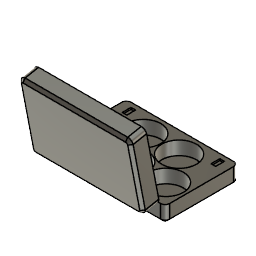
Loupe Case (Autodesk Fusion 360 design; units mm, degrees)
Autodesk Fusion 360 part; units mm, degrees
sketch "Sketch1" plane through (0, 0, 0) normal (0, 0, 1) x (1, 0, 0)
  line L0 (61, 39.8875) -> (-61, 39.8875)
  line L1 (-61, 39.8875) -> (-61, -39.8875)
  line L2 (-61, -39.8875) -> (61, -39.8875)
  line L3 (61, -39.8875) -> (61, 39.8875)
  line L4 (61, 39.8875) -> (-61, -39.8875) construction
  line L5 (-61, 39.8875) -> (61, -39.8875) construction
  line L6 (-71.3663, 44.8875) -> (78.0127, 44.8875) construction
  line L7 (61, 49.8875) -> (-61, 49.8875)
  line L8 (-61, 49.8875) -> (-61, 129.6625)
  line L9 (-61, 129.6625) -> (61, 129.6625)
  line L10 (61, 129.6625) -> (61, 49.8875)
  circle A0 centre (-39, 16.8875) radius 19
  line L11 (0, 0) -> (0, -7.9518) construction
  circle A1 centre (0, 16.8875) radius 19
  circle A2 centre (39, 16.8875) radius 19
  circle A3 centre (-19.5, -16.8875) radius 19
  line L12 (-39, 16.8875) -> (-19.5, -16.8875) construction
  line L13 (-39, 16.8875) -> (-33.2699, 16.8875) construction
  circle A4 centre (19.5, -16.8875) radius 19
  circle A5 centre (19.5, 106.6625) radius 19
  circle A6 centre (-19.5, 106.6625) radius 19
  circle A7 centre (39, 72.8875) radius 19
  circle A8 centre (0, 72.8875) radius 19
  circle A9 centre (-39, 72.8875) radius 19
  dimension "d2" = 79.775
  dimension "d3" = 10
  dimension "d6" = 38
  dimension "d10" = 39
  dimension "d11" = 0
  dimension "d12" = 3
  dimension "d13" = 1
  dimension "d15" = 4
  dimension "d17" = 60
  dimension "d18" = 1
  dimension "d19" = 4
  constraint horizontal L0
  constraint perpendicular L0 L1
  constraint parallel L0 L2
  constraint parallel L1 L3
  constraint coincident L4 L11.start
  constraint coincident L5 L11.start
  constraint coincident L11.start origin
  constraint parallel L0 L6
  constraint symmetric L0.start L6 L7.start
  constraint symmetric L0.end L6 L7.end
  constraint symmetric L1.end L6 L8.end
  constraint symmetric L2.end L6 L9.end
  constraint vertical L11
  constraint vertical L11.start A1.centre
  constraint equal A0 A3
  constraint coincident A0.centre L12.start
  constraint horizontal L13
  constraint coincident A3.centre L12.end
  constraint symmetric L11 A3 A4
  constraint symmetric L6 A0 A9
  constraint symmetric L6 A1 A8
  constraint symmetric L6 A2 A7
  constraint symmetric L6 A3 A6
  constraint symmetric L6 A4 A5
  measures "d2" distance of L0.end L1.end
  measures "d3" distance of L0 L7
  measures "d6" diameter of A0
  measures "d12" distance of L1 A0
  measures "d13" distance of A0 A1
  measures "d15" distance of L0 A0
  measures "d17" angle of L12 L13
  measures "d18" distance of A0 A3
  measures "d19" distance of L2 A3
extrude "Extrude1" add sketch "Sketch1" along normal blind 18 contours L0 L1 L2 L3 | L7 L8 L9 L10 | A0 | A1 | A2 | A3 | A4 | A5 | A6 | A7 | A8 | A9 makes body 1 at (-20.3333, 103.0708, 0) makes body 2 at (-20.3333, 13.2958, 0)
extrude "Extrude2" cut sketch "Sketch1" against normal blind 15 from surface at 18 contours A0 | A1 | A2 | A3 | A4 | A5 | A6 | A7 | A8 | A9 bodies 1 2
sketch "Sketch2" plane through (61, 0, 0) normal (1, 0, 0) x (0, 1, 0)
  line L0 (-39.8875, 0) -> (39.8875, 0)
  line L1 (39.8875, 0) -> (39.8875, 18)
  line L2 (39.8875, 18) -> (-39.8875, 18)
  line L3 (-39.8875, 18) -> (-39.8875, 0)
  line L4 (39.8875, 0) -> (39.8875, 18)
  line L5 (39.8875, 18) -> (39.8875, 0)
  line L6 (49.8875, 0) -> (49.8875, 18)
  line L7 (49.8875, 18) -> (49.8875, 0)
  line L8 (39.8875, 7.3431) -> (47.7159, 15.1716)
  line L9 (49.8875, 7.3431) -> (42.0591, 15.1716)
  line L10 (39.8875, 18) -> (49.8875, 18) construction
  circle A0 centre (44.8875, 18) radius 4
  line L11 (39.8875, 18) -> (40.8875, 18)
  line L12 (49.8875, 18) -> (48.8875, 18)
  dimension "d23" = 135
  dimension "d24" = 135
  dimension "d25" = 1
  constraint coincident L5 L8.start
  constraint coincident L6 L9.start
  constraint coincident L1.end L2.start
  constraint coincident L6.end L7.start
  constraint midpoint L10 A0.centre
  constraint coincident L8.end A0
  constraint tangent L8 A0
  constraint coincident L9.end A0
  constraint tangent L9 A0
  constraint coincident A0 L11.end
  constraint coincident L10 L11.end
  constraint coincident A0 L12.end
  constraint coincident L10 L12.end
  measures "d23" angle of L5 L8
  measures "d24" angle of L6 L9
  measures "d25" distance of L1.end A0
extrude "Extrude3" add sketch "Sketch2" against normal blind 12 from surface at -15 contours L1 L4 L5 L8 L9 A0 L11 | L8 L9 A0 | A0 bodies 2
extrude "Extrude4" add sketch "Sketch2" against normal blind 12 from surface at -27.4 contours L8 L9 A0 | L6 L7 L8 L9 A0 L12 | A0 bodies 1
ref_plane "WorkPlane2" through (38.539, 44.8875, 18) normal (0, 0, 1) x (-1, 0, 0)
sketch "Sketch3" plane through (0, 0, 18) normal (0, 0, 1) x (1, 0, 0)
  line L0 (34, 48.8875) -> (34, 40.8875)
  line L1 (33.6, 40.8875) -> (33.6, 48.8875)
  line L2 (34, 41.8875) -> (37, 44.8875)
  line L3 (33.6, 41.8875) -> (36.6, 44.8875)
  line L4 (53.461, 44.8875) -> (23.617, 44.8875)
  dimension "d33" = 45
  dimension "d34" = 0.4
  dimension "d35" = 1
  constraint coincident L1 L3.start
  constraint coincident L0 L2.start
  constraint parallel L2 L3
  constraint coincident L2.end L4
  constraint coincident L3.end L4
  measures "d33" angle of L3 L4
  measures "d34" distance of L2.end L3.end
  measures "d35" distance of L0.end L2.start
revolve "Revolve1" cut sketch "Sketch3" angle 360 about axis through (53.461, 44.8875, 18) along (-1, 0, 0) contours L0 L3 L4 | L0 L2 L3 L4 bodies 2
revolve "Revolve2" add sketch "Sketch3" angle 360 about axis through (53.461, 44.8875, 18) along (-1, 0, 0) contours L0 L3 L4 | L0 L1 L3 L4 bodies 1
mirror "Mirror1" about plane through (0, 0, 0) normal (1, 0, 0) of "Extrude3", "Extrude4", "Revolve1", "Revolve2"
fillet "Fillet1" radius 5 12 edges at (61, 49.8875, 9) (61, 129.6625, 9) (-61, 129.6625, 9) (-61, 49.8875, 9) (21.6, 49.8875, 12.6716) (-21.6, 49.8875, 12.6716) (-61, -39.8875, 9) (61, -39.8875, 9) (61, 39.8875, 9) (-61, 39.8875, 9) (46, 39.8875, 12.6716) (-46, 39.8875, 12.6716) on bodies 1 2
chamfer "Chamfer1" distance 3 angle 45 16 edges at (0, -39.8875, 0) (59.5355, -38.423, 0) (61, 0, 0) (59.5355, 38.423, 0) (0, 39.8875, 0) (-59.5355, 38.423, 0) (-61, 0, 0) (-59.5355, -38.423, 0) (0, 49.8875, 0) (-59.5355, 51.352, 0) (-61, 89.775, 0) (-59.5355, 128.198, 0) (0, 129.6625, 0) (59.5355, 128.198, 0) (61, 89.775, 0) (59.5355, 51.352, 0) on bodies 1 2
sketch "Sketch4" plane through (0, 0, 18) normal (0, 0, 1) x (-1, 0, 0)
  arc A0 (56, -39.8875) -> (61, -34.8875) centre (56, -34.8875) ccw
  line L0 (61, -34.8875) -> (61, 34.8875)
  arc A1 (61, 34.8875) -> (56, 39.8875) centre (56, 34.8875) ccw
  line L1 (56, 39.8875) -> (-56, 39.8875)
  arc A2 (-56, 39.8875) -> (-61, 34.8875) centre (-56, 34.8875) ccw
  line L2 (-61, 34.8875) -> (-61, -34.8875)
  arc A3 (-61, -34.8875) -> (-56, -39.8875) centre (-56, -34.8875) ccw
  line L3 (-56, -39.8875) -> (-51, -39.8875)
  arc A4 (-48, -40.8875) -> (-51, -39.8875) centre (-51, -44.8875) ccw
  line L4 (-48, -40.8875) -> (-34, -40.8875)
  line L5 (-34, -40.8875) -> (-34, -39.8875)
  line L6 (-34, -39.8875) -> (34, -39.8875)
  line L7 (34, -39.8875) -> (34, -40.8875)
  line L8 (34, -40.8875) -> (48, -40.8875)
  arc A5 (51, -39.8875) -> (48, -40.8875) centre (51, -44.8875) ccw
  line L9 (51, -39.8875) -> (56, -39.8875)
  circle A6 centre (0, -16.8875) radius 19
  circle A7 centre (19.5, 16.8875) radius 19
  circle A8 centre (39, -16.8875) radius 19
  circle A9 centre (-39, -16.8875) radius 19
  circle A10 centre (-19.5, 16.8875) radius 19
  line L10 (51, 25.3875) -> (46, 25.3875)
  line L11 (46, 25.3875) -> (46, 34.8875)
  line L12 (46, 34.8875) -> (51, 34.8875)
  line L13 (51, 34.8875) -> (51, 25.3875)
  line L14 (-53.461, -44.8875) -> (-23.617, -44.8875)
  line L15 (51, -124.6625) -> (51, -115.1625)
  line L16 (46, -124.6625) -> (51, -124.6625)
  line L17 (46, -115.1625) -> (46, -124.6625)
  line L18 (51, -115.1625) -> (46, -115.1625)
  dimension "d43" = 5
  dimension "d44" = 9.5
  dimension "d48" = 5
  dimension "d49" = 10
  constraint horizontal L10
  constraint vertical L11
  constraint horizontal L12
  constraint vertical L13
  constraint symmetric L10.start L14 L15.end
  constraint symmetric L10.end L14 L17.start
  constraint symmetric L11.end L14 L16.start
  constraint symmetric L12.end L14 L15.start
  measures "d43" distance of L10.start L10.end
  measures "d44" distance of L10.start L12.end
  measures "d48" distance of L1 L12
  measures "d49" distance of L0 L13
extrude "Extrude5" cut sketch "Sketch4" against normal blind 2 contours L10 L11 L12 L13 | L15 L16 L17 L18 bodies 1 2
mirror "Mirror2" about plane through (0, 0, 0) normal (1, 0, 0) of "Extrude5"
copy_body "Body->Comp1" bodies 1 removing the originals makes body 3 in component "Top"
copy_body "Body->Comp2" bodies 2 removing the originals makes body 4 in component "Bottom"
move_face "OffsetFaces1" offset -0.2 1 faces at (45.0764, 103.1891, 18) on bodies 3 in component "Top"
move_face "OffsetFaces1'" [no effect] in component "Bottom"
ref_plane "WorkPlane3" through (36.4183, 44.8875, 22) normal (0, 0, 1) x (0, -1, 0)
sketch "Sketch5" plane through (0, 0, 22) normal (0, 0, 1) x (1, 0, 0)
  line L0 (-61, 124.6625) -> (61, 124.6625)
  line L1 (61, 124.6625) -> (61, -34.8875)
  line L2 (61, -34.8875) -> (-61, -34.8875)
  line L3 (-61, -34.8875) -> (-61, 124.6625)
  line L4 (-61, 124.6625) -> (-61, 54.8875)
  line L5 (-61, 54.8875) -> (-61, 124.6625)
  line L6 (61, -34.8875) -> (61, 34.8875)
  line L7 (61, 34.8875) -> (61, -34.8875)
  constraint horizontal L0
  constraint vertical L1
  constraint horizontal L2
  constraint vertical L3
  constraint coincident L1.end L2.start
  constraint coincident L0.start L3.end
extrude "Extrude1'" cut sketch "Sketch5" against normal blind 0.4 bodies 3 in component "Top"
extrude "Extrude1''" cut sketch "Sketch5" against normal blind 0.4 bodies 4 in component "Bottom"
component "Top" placed x (1, 0, 0) y (0, 1, 0) z (0, 0, 1) at (0, 0, 0)
component "Bottom" placed x (1, 0, 0) y (0, 1, 0) z (0, 0, 1) at (0, 0, 0)
named bodies: "Top", "Bottom"
